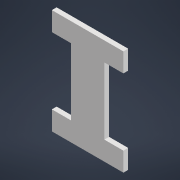
# Autodesk Inventor part: Base
Saved by Autodesk Inventor 2021 (Build 250183000, 183)
## iProperties
Created: 2021-11-22
Part Number: Base
Material: Polypropylene
Document SubType Name: Modeling
Designer: techv
Mass: 196.108 g
Surface Area: 526.32 cm^2
Volume: 218.14 cm^3
Density: 0.899 g/cm^3
Appearance: Smooth - Ash
Author: techv
Autodesk Inventor part; units mm, degrees
ref_plane "YZ Plane" through (0, 0, 0) normal (1, 0, 0) x (0, 1, 0)
ref_plane "XZ Plane" through (0, 0, 0) normal (0, 1, 0) x (-1, 0, 0)
ref_plane "XY Plane" through (0, 0, 0) normal (0, 0, 1) x (1, 0, 0)
sketch "Sketch1" plane through (0, 0, 0) normal (0, 0, 1) x (1, 0, 0)
  line L0 (-65, 100.1) -> (65, 100.1) construction
  line L1 (65, 100.1) -> (65, -100.1) construction
  line L2 (65, -100.1) -> (-65, -100.1) construction
  line L3 (-65, -100.1) -> (-65, 100.1) construction
  line L4 (-65, 100.1) -> (65, -100.1) construction
  line L5 (65, 100.1) -> (-65, -100.1) construction
  line L6 (-75, 110.1) -> (75, 110.1)
  line L7 (75, 110.1) -> (75, -110.1) construction
  line L8 (75, -110.1) -> (-75, -110.1)
  line L9 (-75, -110.1) -> (-75, 110.1) construction
  line L10 (-75, 110.1) -> (75, -110.1) construction
  line L11 (75, 110.1) -> (-75, -110.1) construction
  line L12 (75, 110.1) -> (75, 70.1)
  line L13 (75, 70.1) -> (35, 70.1)
  line L14 (35, 70.1) -> (35, -70.1)
  line L15 (35, -70.1) -> (75, -70.1)
  line L16 (75, -110.1) -> (75, -70.1)
  line L17 (0, 110.1) -> (0, -110.1) construction
  line L18 (-75, 110.1) -> (-75, -110.1) construction
  line L19 (-75, 110.1) -> (-75, 70.1)
  line L20 (-75, 70.1) -> (-35, 70.1)
  line L21 (-35, 70.1) -> (-35, -70.1)
  line L22 (-35, -70.1) -> (-75, -70.1)
  line L23 (-75, -110.1) -> (-75, -70.1)
  point P0 (0, 0)
  dimension "d0" = 130
  dimension "d1" = 200.2
  dimension "d2" = 150
  dimension "d3" = 220.2
  dimension "d4" = 40
  dimension "d5" = 40
  dimension "d6" = 140.2
  dimension "d7" = 90
  constraints: 48 end point, 6 midpoint, 5 perpendicular, 4 parallel, 4 point on line, 4 symmetric about line, 2 collinear, 2 horizontal
  measures "d0" distance of L1.end L2.end
  measures "d1" distance of L0.end L1.end
  measures "d2" distance of L7.end L8.end
  measures "d3" distance of L6.end L7.end
  measures "d4" distance of L6.end L12.end
  measures "d5" distance of L12.end L13.end
  measures "d6" distance of L13.end L14.end
  measures "d7" angle of L14 L13
extrude "Extrusion1" add sketch "Sketch1" along normal blind 10
sketch "Sketch2" plane through (0, 0, 10) normal (0, 0, 1) x (1, 0, 0)
  line L0 (65, 100.1) -> (-65, -100.1) construction
  line L1 (-65, 100.1) -> (65, -100.1) construction
  circle A0 centre (65, 100.1) radius 5
  circle A1 centre (-65, 100.1) radius 5
  circle A2 centre (-65, -100.1) radius 5
  circle A3 centre (65, -100.1) radius 5
  point P0 (0, 0)
  dimension "d10" = 10
  dimension "d11" = 10
  dimension "d12" = 10
  dimension "d13" = 10
  constraints: 4 centre point, 4 coincident
  measures "d10" diameter of A0
  measures "d11" diameter of A1
  measures "d12" diameter of A2
  measures "d13" diameter of A3
equation "\"d1\" = 1.54 * d0"
equation "\"d11\" = d10"
equation "\"d12\" = d10"
body "Solid1"
